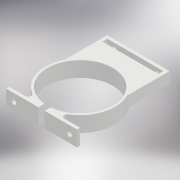
# Autodesk Inventor part: OmegaRing
Saved by Autodesk Inventor 2018.2 (Build 222227000, 227)
## iProperties
Created: 2018-03-27
Part Number: OmegaRing
Material: ABS Plastic
Document SubType Name: Modeling
Designer: mansu
Density: 1.06 g/cm^3
Appearance: Smooth - White
Author: mansu
Autodesk Inventor part; units mm, degrees
ref_plane "YZ Plane" through (0, 0, 0) normal (1, 0, 0) x (0, 1, 0)
ref_plane "XZ Plane" through (0, 0, 0) normal (0, 1, 0) x (-1, 0, 0)
ref_plane "XY Plane" through (0, 0, 0) normal (0, 0, 1) x (1, 0, 0)
sketch "Sketch1" plane through (0, 0, 0) normal (0, 0, 1) x (1, 0, 0)
  circle A0 centre (0, 0) radius 21.15 construction
  line L0 (-18, -25) -> (18, -25) construction
  line L1 (-18, -25) -> (-18, -38.1522) construction
  line L2 (18, -25) -> (18, -38.1522) construction
  line L3 (-23, -23) -> (-23, -25)
  line L4 (-23, -25) -> (-2, -25)
  line L5 (-2, -21.0552) -> (-2, -25)
  line L6 (2, -21.0552) -> (2, -25)
  line L7 (2, -25) -> (23, -25)
  line L8 (23, -25) -> (23, -23)
  line L9 (23, -23) -> (12.7162, -23)
  line L10 (-23, -23) -> (-12.7162, -23)
  arc A1 (11.6803, -19.2892) -> (-11.6803, -19.2892) centre (0, 0) ccw
  arc A2 (2, -21.0552) -> (-2, -21.0552) centre (0, 0) ccw
  arc A3 (11.6803, -19.2892) -> (12.7162, -23) centre (12.7162, -21) ccw
  arc A4 (-12.7162, -23) -> (-11.6803, -19.2892) centre (-12.7162, -21) ccw
  point P0 (0, -25)
  dimension "d13" = 42.3
  dimension "d1" = 25
  dimension "d2" = 36
  dimension "d3" = 2
  dimension "d4" = 1.4
  dimension "d5" = 5
  dimension "d6" = 2
  dimension "d7" = 4
  constraints: 22 end point, 8 point on circle, 5 perpendicular, 4 centre point, 4 point on line, 4 tangent, 2 horizontal, 2 horizontal alignment, 2 vertical, 1 coincident, 1 collinear, 1 concentric, 1 equal radius, 1 midpoint, 1 vertical alignment, 4 other
  measures "d1" distance from line of point (0, 0) L0
  measures "d2" distance of L0.start L0.end
  measures "d3" distance of L7.end L8.end
  measures "d5" distance between parallel lines of L1 L3
  measures "d6" radius of A3
  measures "d7" distance between parallel lines of L5 L6
extrude "Extrusion1" add sketch "Sketch1" along normal blind 10
sketch "Sketch2" plane through (2, -25, 0) normal (0, -1, 0) x (1, 0, 0)
  circle A0 centre (16, 5) radius 1.5
  line L0 (21, 0) -> (21, 10) projected
  point P0 (-2, 0)
  point P1 (16, 0)
  point P2 (16, 0)
  point P3 (16, 0)
  point P4 (21, 5)
  dimension "d10" = 3
  constraints: 1 centre point, 1 horizontal alignment, 1 midpoint, 1 vertical alignment
  measures "d10" diameter of A0
extrude "Extrusion2" cut sketch "Sketch2" against normal up to surface (2 mm away)
mirror "Mirror1" about plane through (0, 0, 0) normal (1, 0, 0) of "Extrusion2"
sketch "Sketch3" plane through (0, 0, 10) normal (0, 0, 1) x (1, 0, 0)
  arc A0 (21.9303, 5.25) -> (-21.9303, 5.25) centre (0, 0) ccw projected
  line L0 (-18.15, 35.75) -> (18.15, 35.75)
  line L1 (18.15, 35.75) -> (18.15, 32.55)
  line L2 (18.15, 32.55) -> (-18.15, 32.55)
  line L3 (-18.15, 32.55) -> (-18.15, 35.75)
  line L4 (-20.15, 37.75) -> (20.15, 37.75)
  line L5 (20.15, 37.75) -> (20.15, 10.1232)
  arc A1 (11.6803, -19.2892) -> (-11.6803, -19.2892) centre (0, 0) ccw projected
  line L6 (-20.15, 37.75) -> (-20.15, 10.1232)
  point P0 (0, 35.75)
  dimension "d14" = 3.2
  dimension "d15" = 36.3
  dimension "d16" = 10
  dimension "d17" = 2
  dimension "d18" = 2
  dimension "d19" = 2
  constraints: 14 end point, 2 horizontal, 2 parallel, 2 perpendicular, 2 point on circle, 1 midpoint, 1 vertical, 1 vertical alignment
  measures "d14" distance of L0.end L1.end
  measures "d15" distance of L0.start L0.end
  measures "d16" distance edge to line of A0 L2
  measures "d17" distance between parallel lines of L0 L4
  measures "d18" distance between parallel lines of L3 L6
  measures "d19" distance between parallel lines of L1 L5
extrude "Extrusion3" add sketch "Sketch3" against normal blind 7
sketch "Sketch4" plane through (-20.15, 37.75, 10) normal (0, 1, 0) x (1, 0, 0)
  circle A0 centre (34.15, 3.5) radius 1.5
  circle A1 centre (6.15, 3.5) radius 1.5
  line L0 (34.15, 3.5) -> (6.15, 3.5) construction
  line L1 (0, 7) -> (40.3, 7) construction
  line L2 (0, 0) -> (0, 7) projected
  point P0 (20.15, 10)
  point P1 (20.15, 3.5)
  point P2 (20.15, 7)
  point P3 (0, 3.5)
  dimension "d22" = 3
  dimension "d23" = 3
  dimension "d24" = 28
  constraints: 2 centre point, 2 end point, 2 horizontal alignment, 2 midpoint, 1 horizontal, 1 vertical alignment, 2 other
  measures "d22" diameter of A0
  measures "d23" diameter of A1
  measures "d24" distance of L0.start L0.end
extrude "Extrusion4" cut sketch "Sketch4" against normal blind 12
body "Solid1"
